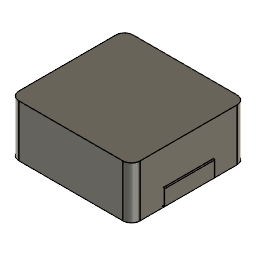
L0630电感 (Autodesk Fusion 360 design; units mm, degrees)
Autodesk Fusion 360 part; units mm, degrees
sketch "草图1" plane through (0, 0, 0) normal (0, 0, 1) x (1, 0, 0)
  line L0 (-3, -3.3) -> (3, -3.3)
  line L1 (3.5, -2.8) -> (3.5, 2.8)
  line L2 (3, 3.3) -> (-3, 3.3)
  line L3 (-3.5, 2.8) -> (-3.5, -2.8)
  line L4 (-3.5, -3.3) -> (3.5, 3.3) construction
  line L5 (3.5, -3.3) -> (-3.5, 3.3) construction
  arc A0 (-3, 3.3) -> (-3.5, 2.8) centre (-3, 2.8) ccw
  arc A1 (3.5, 2.8) -> (3, 3.3) centre (3, 2.8) ccw
  arc A2 (3, -3.3) -> (3.5, -2.8) centre (3, -2.8) ccw
  arc A3 (-3.5, -2.8) -> (-3, -3.3) centre (-3, -2.8) ccw
  dimension "d1" = 6.6
  dimension "d2" = 7
  dimension "d3" = 0.5
  dimension "d4" = 0.5
  constraint horizontal L0
  constraint perpendicular L0 L1
  constraint parallel L0 L2
  constraint parallel L1 L3
  constraint coincident L4 origin
  constraint coincident L5 origin
  constraint coincident L5.end L2
  constraint coincident L5.end L3
  constraint tangent L2 A0
  constraint tangent L3 A0
  constraint coincident L4.end L2
  constraint coincident L4.end L1
  constraint tangent L2 A1
  constraint tangent L1 A1
  constraint coincident L5.start L1
  constraint coincident L5.start L0
  constraint tangent L1 A2
  constraint tangent L0 A2
  constraint equal A1 A2
  constraint coincident L4.start L0
  constraint coincident L4.start L3
  constraint tangent L0 A3
  constraint tangent L3 A3
  constraint equal A1 A3
  measures "d1" distance of L5.start L4.end
  measures "d2" distance of L4.start L5.start
  measures "d3" radius of A0
  measures "d4" radius of A1
extrude "拉伸1" add sketch "草图1" along normal blind 3 makes body 1
sketch "草图2" plane through (3.5, 0, 0) normal (1, 0, 0) x (0, 1, 0)
  line L0 (-2.8, 0) -> (2.8, 0)
  line L1 (2.8, 0) -> (2.8, 3)
  line L2 (2.8, 3) -> (-2.8, 3)
  line L3 (-2.8, 3) -> (-2.8, 0)
  line L4 (-1.5, 1) -> (1.5, 1)
  line L5 (1.5, 1) -> (1.5, 0)
  line L6 (1.5, 0) -> (-1.5, 0)
  line L7 (-1.5, 0) -> (-1.5, 1)
  dimension "d7" = 3
  dimension "d8" = 1
  dimension "d9" = 1.5
  constraint horizontal L4
  constraint vertical L5
  constraint horizontal L6
  constraint vertical L7
  constraint coincident L0 L5.end
  measures "d7" distance of L5.end L6.end
  measures "d8" distance of L4.end L5.end
  measures "d9" distance of origin L5.end
sketch "草图3" plane through (0, 0, 0) normal (0, 0, -1) x (1, 0, 0)
  arc A0 (-3, 3.3) -> (-3.5, 2.8) centre (-3, 2.8) ccw
  line L0 (-3.5, 2.8) -> (-3.5, -2.8)
  arc A1 (-3.5, -2.8) -> (-3, -3.3) centre (-3, -2.8) ccw
  line L1 (-3, -3.3) -> (3, -3.3)
  arc A2 (3, -3.3) -> (3.5, -2.8) centre (3, -2.8) ccw
  line L2 (3.5, -2.8) -> (3.5, 2.8)
  arc A3 (3.5, 2.8) -> (3, 3.3) centre (3, 2.8) ccw
  line L3 (3, 3.3) -> (-3, 3.3)
  line L4 (3.5, 1.5) -> (2, 1.5)
  line L5 (2, 1.5) -> (2, -1.5)
  line L6 (2, -1.5) -> (3.5, -1.5)
  line L7 (3.5, -1.5) -> (3.5, 1.5)
  dimension "d10" = 1.5
  dimension "d11" = 3
  dimension "d12" = 1.5
  constraint horizontal L4
  constraint vertical L5
  constraint horizontal L6
  constraint vertical L7
  constraint coincident L2 L4.start
  measures "d10" distance of L4.start L4.end
  measures "d11" distance of L4 L6
  measures "d12" vertical distance of origin L6.end
sketch "草图4" plane through (3.5, 0, 0) normal (1, 0, 0) x (0, 1, 0)
extrude "拉伸2" cut sketch "草图3" against normal blind 0.1 contours L2 L4 L5 L6 L7 bodies 1
sketch "草图5" plane through (0, 0, 0) normal (0, 0, 1) x (1, 0, 0)
  line L0 (-3.5, 1.5) -> (-2, 1.5)
  line L1 (-2, 1.5) -> (-2, -1.5)
  line L2 (-2, -1.5) -> (-3.5, -1.5)
  line L3 (-3.5, -1.5) -> (-3.5, 1.5)
  dimension "d15" = 1.5
  dimension "d16" = 3
  dimension "d17" = 1.5
  dimension "d18" = 3.5
  constraint horizontal L0
  constraint vertical L1
  constraint horizontal L2
  constraint vertical L3
  measures "d15" distance of L0.start L0.end
  measures "d16" distance of L0.end L1.end
  measures "d17" vertical distance of origin L1.end
  measures "d18" distance of origin L3
extrude "拉伸3" cut sketch "草图5" along normal blind 0.1 bodies 1
sketch "草图6" plane through (-3.5, 0, 0) normal (-1, 0, 0) x (0, -1, 0)
  line L0 (1.5, 0.1) -> (1.5, 0)
  line L1 (1.5, 0) -> (2.8, 0)
  line L2 (2.8, 0) -> (2.8, 3)
  line L3 (2.8, 3) -> (-2.8, 3)
  line L4 (-2.8, 3) -> (-2.8, 0)
  line L5 (-2.8, 0) -> (-1.5, 0)
  line L6 (-1.5, 0) -> (-1.5, 0.1)
  line L7 (-1.5, 0.1) -> (1.5, 0.1)
  line L8 (-1.5, 0) -> (1.5, 0)
  line L9 (1.5, 0) -> (1.5, 1)
  line L10 (1.5, 1) -> (-1.5, 1)
  line L11 (-1.5, 1) -> (-1.5, 0)
  dimension "d21" = 3
  dimension "d22" = 1
  constraint horizontal L8
  constraint vertical L9
  constraint horizontal L10
  constraint vertical L11
  constraint coincident L5.end L6.start
  measures "d21" distance of L9.end L10.end
  measures "d22" distance of L0.end L9.end
extrude "拉伸4" cut sketch "草图6" against normal blind 0.1 contours L7 L9 L10 L11 bodies 1
sketch "草图7" plane through (0, 1.5, 0) normal (0, -1, 0) x (1, 0, 0)
  line L0 (-3.5, 0) -> (-2, 0)
  line L1 (-2, 0) -> (-2, 0.1)
  line L2 (-2, 0.1) -> (-3.4, 0.1)
  line L3 (-3.4, 0.1) -> (-3.4, 1)
  line L4 (-3.4, 1) -> (-3.5, 1)
  line L5 (-3.5, 1) -> (-3.5, 0)
  line L6 (-3.4, 1) -> (-3.5, 1)
  line L7 (-3.55, 0.95) -> (-3.55, 0.05)
  line L8 (-3.5, 0) -> (-2.05, 0)
  line L9 (-2, 0.1) -> (-2, 0.05)
  line L10 (-2, 0.1) -> (-3.4, 0.1)
  line L11 (-3.4, 0.1) -> (-3.4, 1)
  arc A0 (-3.5, 1) -> (-3.55, 0.95) centre (-3.5, 0.95) ccw
  arc A1 (-3.55, 0.05) -> (-3.5, 0) centre (-3.5, 0.05) ccw
  arc A2 (-2.05, 0) -> (-2, 0.05) centre (-2.05, 0.05) ccw
  dimension "d25" = 0.05
  constraint coincident L3.end L4.start
  constraint perpendicular L3 L6
  constraint perpendicular L6 L7
  constraint perpendicular L1 L8
  constraint coincident L1.end L2.start
  constraint coincident L2.end L3.start
  constraint tangent L6 A0
  constraint tangent L7 A0
  constraint tangent L7 A1
  constraint tangent L8 A1
  constraint equal A0 A1
  constraint tangent L8 A2
  constraint tangent L9 A2
  constraint equal A0 A2
  measures "d25" radius of A0
extrude "拉伸5" add sketch "草图7" along normal blind 2.9 separate body contours L0 L1 L2 L3 L4 L5 L6 L8 L9 L10 L11 A2 | L5 L7 A0 A1 makes body 2
move_body "移动1" bodies 2 to x (1, 0, 0) y (0, 1, 0) z (0, 0, 1) at (0, -0.05, 0)
copy_body "复制和粘贴实体1" bodies 2 makes body 3
move_body "移动2" bodies 3 to x (1, 0, 0) y (0, 1, 0) z (0, 0, 1) at (7.4, 0, 0)
move_body "移动3" bodies 3 to x (-1, 0, 0) y (0, -1, 0) z (0, 0, 1) at (9.25, 0, 0)
move_body "移动4" bodies 3 to x (1, 0, 0) y (0, 1, 0) z (0, 0, 1) at (-1.85, 0, 0)
